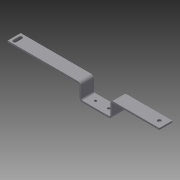
# Autodesk Inventor part: Cylinder Mount
Saved by Autodesk Inventor 2013 (Build 170138000, 138)
## iProperties
Created: 2013-01-26
Part Number: Cylinder Mount
Material: Generic
Document SubType Name: Sheet Metal
Designer: actoennies
Density: 1 g/cm^3
Sheet Metal Rule: Default
Mass: 27.1604 g
Surface Area: 197.649 cm^2
Volume: 27.1604 cm^3
Author: actoennies
Autodesk Inventor part; units mm, degrees
ref_plane "YZ Plane" through (0, 0, 0) normal (1, 0, 0) x (0, 1, 0)
ref_plane "XZ Plane" through (0, 0, 0) normal (0, 1, 0) x (-1, 0, 0)
ref_plane "XY Plane" through (0, 0, 0) normal (0, 0, 1) x (1, 0, 0)
sketch "Sketch1" plane through (0, 0, 0) normal (0, 1, 0) x (-1, 0, 0)
  line L0 (0, 0) -> (0, 25.4)
  line L1 (0, 25.4) -> (50.8, 25.4)
  line L2 (50.8, 25.4) -> (50.8, 0)
  line L3 (50.8, 0) -> (0, 0)
  dimension "d0" = 25.4
  dimension "d1" = 50.8
  measures "d0" distance of L0.start L0.end
  measures "d1" distance of L0.end L1.end
extrude "Plate1" add sketch "Sketch1" along normal blind 3.175
sketch "Sketch2" plane through (3.175, 6.35, 0) normal (1, 0, 0) x (0, 1, 0)
  line L0 (0, 25.4) -> (0, 0)
  line L1 (0, 0) -> (19.05, 0)
  line L2 (19.05, 0) -> (19.05, 25.4)
  line L3 (19.05, 25.4) -> (0, 25.4)
  constraints: 6 end point, 1 horizontal, 1 perpendicular, 1 vertical
edge flange "Flange1" height 25.4 angle 90 thickness 3.175 bend radius 3.175 thickness toward (1, 0, 0) relief straight relief width 3.175 relief depth 1.5875 corner gap 3.175 corner form 0 edges at (0, 3.175, 12.7) (-50.8, 3.175, 12.7) wall of the first edge with corners at (3.175, 6.35, 25.4) (3.175, 6.35, 0) (3.175, 25.4, 0) (3.175, 25.4, 25.4)
bend "Bend1"
corner "Corner1"
sketch "Sketch3" plane through (9.525, 28.575, 25.4) normal (0, 1, 0) x (-1, 0, 0)
  line L0 (0, -25.4) -> (0, 0)
  line L1 (0, 0) -> (-88.9, 0)
  line L2 (-88.9, 0) -> (-88.9, -25.4)
  line L3 (-88.9, -25.4) -> (0, -25.4)
  constraints: 6 end point, 1 horizontal, 1 perpendicular, 1 vertical
edge flange "Flange2" height 95.25 angle 90 thickness 3.175 bend radius 3.175 thickness toward (0, 1, 0) relief straight relief width 3.175 relief depth 1.5875 edges at (6.35, 25.4, 12.7) wall of the first edge with corners at (9.525, 28.575, 0) (9.525, 28.575, 25.4) (98.425, 28.575, 25.4) (98.425, 28.575, 0)
bend "Bend2"
corner "Corner2"
sketch "Sketch4" plane through (-60.325, 28.575, 0) normal (0, 1, 0) x (-1, 0, 0)
  line L0 (0, 25.4) -> (0, 0)
  line L1 (0, 0) -> (136.525, 0)
  line L2 (136.525, 0) -> (136.525, 25.4)
  line L3 (136.525, 25.4) -> (0, 25.4)
  constraints: 6 end point, 1 horizontal, 1 perpendicular, 1 vertical
edge flange "Flange3" height 142.875 angle 90 thickness 3.175 bend radius 3.175 thickness toward (0, 1, 0) relief straight relief width 3.175 relief depth 1.5875 edges at (-57.15, 25.4, 12.7) wall of the first edge with corners at (-60.325, 28.575, 25.4) (-60.325, 28.575, 0) (-196.85, 28.575, 0) (-196.85, 28.575, 25.4)
bend "Bend3"
corner "Corner3"
sketch "Sketch5" plane through (0, 0, 0) normal (0, -1, 0) x (1, 0, 0)
  line L0 (0, 25.4) -> (-50.8, 25.4) projected
  line L1 (-50.8, 0) -> (0, 0) projected
  circle A0 centre (-38.1, 12.7) radius 2.54
  circle A1 centre (-12.7, 12.7) radius 2.54
  line L2 (-25.4, 25.4) -> (-25.4, 0)
  dimension "d33" = 5.08
  dimension "d34" = 5.08
  dimension "d35" = 25.4
  dimension "d36" = 12.7
  constraints: 2 centre point, 2 end point, 2 midpoint
  measures "d33" diameter of A0
  measures "d34" diameter of A1
  measures "d35" distance of A1.centre A0.centre
  measures "d36" distance from line of A1.centre L2
extrude "Cut1" cut sketch "Sketch5" against normal blind 3.175
sketch "Sketch6" plane through (98.425, 28.575, 0) normal (0, -1, 0) x (1, 0, 0)
  line L0 (0, 0) -> (-88.9, 0) projected
  line L1 (0, 0) -> (0, 25.4) projected
  circle A0 centre (-12.7, 12.7) radius 3.3782
  point P0 (-98.425, 0)
  dimension "d39" = 6.7564
  dimension "d41" = 12.7
  dimension "d42" = 12.7
  constraints: 1 centre point
  measures "d39" diameter of A0
  measures "d41" distance from line of L1 A0.centre
  measures "d42" distance from line of L0 A0.centre
extrude "Cut2" cut sketch "Sketch6" against normal blind 3.175
sketch "Sketch8" plane through (-196.85, 28.575, 0) normal (0, -1, 0) x (1, 0, 0)
  circle A0 centre (7.62, 14.0411) radius 3.3782 projected
  point P0 (196.85, 0)
extrude "Cut4" cut sketch "Sketch8" against normal blind 3.175
sketch "Sketch9" plane through (-196.85, 31.75, 25.4) normal (0, 1, 0) x (1, 0, 0)
  circle A0 centre (7.62, 11.3589) radius 3.3782 projected
  line L0 (136.525, 0) -> (0, 0) projected
  arc A1 (10.9982, 17.7089) -> (4.2418, 17.7089) centre (7.62, 17.7089) ccw
  arc A2 (4.2418, 6.2789) -> (10.9982, 6.2789) centre (7.62, 6.2789) ccw
  line L1 (4.2418, 6.2789) -> (4.2418, 17.7089)
  line L2 (10.9982, 17.7089) -> (10.9982, 6.2789)
  point P0 (196.85, 25.4)
  dimension "d49" = 6.7564
  dimension "d50" = 6.7564
  dimension "d51" = 5.08
  dimension "d52" = 6.35
  constraints: 4 end point, 4 point on circle, 2 centre point, 2 tangent, 1 perpendicular
  measures "d49" diameter of A1
  measures "d50" diameter of A2
  measures "d51" distance of A0.centre A2.centre
  measures "d52" distance of A1.centre A0.centre
extrude "Cut5" cut sketch "Sketch9" against normal blind 3.175 contours L2 A2 L1 A0 | A0 L1 A1 L2
equation "\"d37\" = Thickness"
equation "\"d43\" = Thickness"
equation "\"d47\" = Thickness"
equation "\"d53\" = Thickness"
equation "\"d3\" = BendReliefWidth"
equation "\"d4\" = BendReliefDepth"
equation "\"d5\" = MinimumRemnant"
equation "\"d6\" = BendRadius"
equation "\"d9\" = BendRadius"
equation "\"d10\" = CornerReliefSize"
equation "\"d11\" = GapSize"
equation "\"d12\" = JacobiRadiusSize"
equation "\"d13\" = BendReliefWidth"
equation "\"d14\" = BendReliefDepth"
equation "\"d15\" = MinimumRemnant"
equation "\"d16\" = BendRadius"
equation "\"d19\" = BendRadius"
equation "\"d20\" = CornerReliefSize"
equation "\"d21\" = GapSize"
equation "\"d22\" = JacobiRadiusSize"
equation "\"d23\" = BendReliefWidth"
equation "\"d24\" = BendReliefDepth"
equation "\"d25\" = MinimumRemnant"
equation "\"d26\" = BendRadius"
equation "\"d29\" = BendRadius"
equation "\"d30\" = CornerReliefSize"
equation "\"d31\" = GapSize"
equation "\"d32\" = JacobiRadiusSize"
equation "\"BendRadius\" = Thickness"
equation "\"BendReliefWidth\" = Thickness"
equation "\"BendReliefDepth\" = 0.5 * Thickness"
equation "\"CornerReliefSize\" = 4 * Thickness"
equation "\"MinimumRemnant\" = 2 * Thickness"
equation "\"TransitionRadius\" = BendRadius"
equation "\"JacobiRadiusSize\" = BendRadius"
equation "\"GapSize\" = Thickness"
equation "\"d2\" = BendRadius"
equation "\"Thickness\" = 3.175"
body "Solid1"
